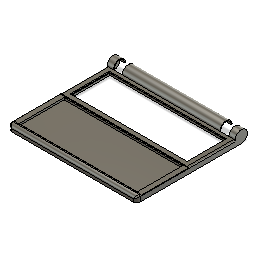
C_case (Autodesk Fusion 360 design; units mm, degrees)
Autodesk Fusion 360 part; units mm, degrees
sketch "Sketch1" plane through (0, 0, 0) normal (0, 1, 0) x (1, 0, 0)
  line L0 (0, 0) -> (230.6, 0)
  line L1 (230.6, 0) -> (230.6, 177.2)
  line L2 (230.6, 177.2) -> (0, 177.2)
  line L3 (0, 177.2) -> (0, 0)
  dimension "d1" = 230.6
  dimension "d2" = 177.2
  constraint horizontal L0
  constraint vertical L1
  constraint horizontal L2
  constraint vertical L3
  constraint coincident L0.start L3.end
  measures "d1" distance of L0.start L0.end
  measures "d2" distance of L0.start L2.end
extrude "Extrude1" add sketch "Sketch1" along normal blind 11 makes body 1
fillet "Fillet3" radius 2.5 2 edges at (230.6, 11, -88.6) (0, 11, -88.6) on bodies 1
sketch "Sketch2" plane through (0, 11, 0) normal (0, 1, 0) x (-1, 0, 0)
  line L0 (-2.5, 0) -> (-228.1, 0)
  line L1 (-228.1, -177.2) -> (-2.5, -177.2)
  line L2 (-9, -10) -> (-221.6, -10)
  line L3 (-221.6, -10) -> (-221.6, -91.1)
  line L4 (-221.6, -91.1) -> (-9, -91.1)
  line L5 (-9, -91.1) -> (-9, -10)
  line L6 (-115.3, -77.3448) -> (-115.3, -22.2714) construction
  line L7 (-228.1, 0) -> (-228.1, -177.2)
  line L8 (-2.5, -177.2) -> (-2.5, 0)
  dimension "d5" = 212.6
  dimension "d6" = 81.1
  dimension "d7" = 10
  constraint horizontal L2
  constraint vertical L3
  constraint horizontal L4
  constraint vertical L5
  constraint perpendicular L1 L6
  constraint symmetric L3 L5 L6
  measures "d5" distance of L3.end L4.end
  measures "d6" distance of L2.start L4.end
  measures "d7" distance of L0 L2
extrude "Extrude2" cut sketch "Sketch2" against normal blind 5 contours L2 L3 L4 L5 bodies 1
sketch "Sketch3" plane through (0, 11, 0) normal (0, 1, 0) x (-1, 0, 0)
  line L0 (-221.6, -10) -> (-9, -10)
  line L1 (-9, -10) -> (-9, -91.1)
  line L2 (-9, -91.1) -> (-221.6, -91.1)
  line L3 (-221.6, -91.1) -> (-221.6, -10)
  line L4 (-2.5, 0) -> (-228.1, 0)
  line L5 (-228.1, -177.2) -> (-2.5, -177.2)
  line L6 (-10.05, -171.2) -> (-220.55, -171.2)
  line L7 (-220.55, -171.2) -> (-220.55, -100.7)
  line L8 (-220.55, -100.7) -> (-10.05, -100.7)
  line L9 (-10.05, -100.7) -> (-10.05, -171.2)
  line L10 (-115.3, -155) -> (-115.3, -110) construction
  line L11 (-228.1, 0) -> (-228.1, -177.2)
  line L12 (-2.5, -177.2) -> (-2.5, 0)
  dimension "d10" = 210.5
  dimension "d11" = 70.5
  dimension "d12" = 6
  constraint horizontal L6
  constraint vertical L7
  constraint horizontal L8
  constraint vertical L9
  constraint vertical L10
  constraint symmetric L7 L9 L10
  measures "d10" distance of L6.start L6.end
  measures "d11" distance of L6.start L8.end
  measures "d12" distance of L5 L6
extrude "Extrude3" cut sketch "Sketch3" against normal blind 1.95 contours L6 L7 L8 L9 bodies 1
sketch "Sketch4" plane through (0, 9.05, 0) normal (0, 1, 0) x (-1, 0, 0)
  line L0 (-10.05, -100.7) -> (-220.55, -100.7)
  line L1 (-220.55, -100.7) -> (-220.55, -171.2)
  line L2 (-220.55, -171.2) -> (-10.05, -171.2)
  line L3 (-10.05, -171.2) -> (-10.05, -100.7)
  line L4 (-11.55, -170.7) -> (-219.05, -170.7)
  line L5 (-219.05, -170.7) -> (-219.05, -101.2)
  line L6 (-219.05, -101.2) -> (-11.55, -101.2)
  line L7 (-11.55, -101.2) -> (-11.55, -170.7)
  dimension "d15" = 0.5
  dimension "d16" = 0.5
  dimension "d17" = 1.5
  dimension "d18" = 1.5
  constraint horizontal L4
  constraint vertical L5
  constraint horizontal L6
  constraint vertical L7
  measures "d15" distance of L2 L4
  measures "d16" distance of L0 L6
  measures "d17" distance of L3 L7
  measures "d18" distance of L1 L5
extrude "Extrude4" cut sketch "Sketch4" against normal blind 4.75 contours L4 L5 L6 L7 bodies 1
sketch "Sketch6" plane through (0, 0, 0) normal (-1, 0, 0) x (0, 0, 1)
  line L0 (-177.2, 0) -> (0, 0)
  line L1 (0, 0) -> (0, 8.5)
  line L2 (-177.2, 8.5) -> (-177.2, 0)
  line L3 (-8, 11) -> (-93, 11)
  line L4 (-93, 11) -> (-93, 9.5)
  line L5 (-93, 9.5) -> (-8, 9.5)
  line L6 (-8, 9.5) -> (-8, 11)
  line L7 (0, 8.5) -> (-177.2, 8.5)
  dimension "d26" = 1.5
  dimension "d27" = 85
  dimension "d28" = 8
  constraint horizontal L3
  constraint vertical L4
  constraint horizontal L5
  constraint vertical L6
  measures "d26" distance of L3.start L5.end
  measures "d27" distance of L3.start L3.end
  measures "d28" distance of L1 L6
extrude "Extrude6" cut sketch "Sketch6" against normal through all contours L3 L4 L5 L6 bodies 1
sketch "Sketch7" plane through (0, 6, 0) normal (0, 1, 0) x (-1, 0, 0)
  line L0 (-9, -91.1) -> (-9, -10)
  line L1 (-9, -10) -> (-221.6, -10)
  line L2 (-221.6, -10) -> (-221.6, -91.1)
  line L3 (-221.6, -91.1) -> (-9, -91.1)
  line L4 (-54, -11.5) -> (-92, -11.5)
  line L5 (-92, -11.5) -> (-92, -23.5)
  line L6 (-92, -23.5) -> (-54, -23.5)
  line L7 (-54, -23.5) -> (-54, -11.5)
  dimension "d32" = 38
  dimension "d33" = 12
  dimension "d34" = 45
  dimension "d35" = 1.5
  constraint horizontal L4
  constraint vertical L5
  constraint horizontal L6
  constraint vertical L7
  measures "d32" distance of L5.end L6.end
  measures "d33" distance of L4.end L5.end
  measures "d34" distance of L0 L7
  measures "d35" distance of L1 L4
sketch "Sketch8" plane through (0, 0, 0) normal (-1, 0, 0) x (0, 0, 1)
  line L0 (-177.2, 8.5) -> (-177.2, 0)
  line L1 (-177.2, 0) -> (0, 0)
  line L2 (0, 0) -> (0, 8.5)
  circle A0 centre (-188.2, 11) radius 11
  circle A1 centre (-188.2, 11) radius 9.5
  line L3 (-177.2, 0) -> (-188.2, 0)
  line L4 (0, 8.5) -> (-177.2, 8.5)
  line L5 (-177.2, 0) -> (-177.2, 11)
  dimension "d36" = 22
  dimension "d37" = 19
  constraint tangent L0 A0
  constraint concentric A0 A1
  constraint coincident L0.end L1.start
  constraint coincident A0 L3.end
  constraint tangent A0 L3
  constraint parallel L1 L3
  constraint coincident A0 L5.end
  constraint tangent A0 L5
  measures "d36" diameter of A0
  measures "d37" diameter of A1
extrude "Extrude7" add sketch "Sketch8" against normal blind 230.6 separate body contours A0 makes body 2
extrude "Extrude8" add sketch "Sketch8" against normal blind 1.5 contours L0 A0 L3 L5 | A0 | A1 bodies 2 1
sketch "Sketch9" plane through (230.6, 0, 0) normal (1, 0, 0) x (0, 0, -1)
  circle A0 centre (188.2, 11) radius 9.5
  circle A1 centre (188.2, 11) radius 11
  circle A2 centre (188.2, 11) radius 11
  line L0 (177.2, 0) -> (188.2, 0)
  line L1 (177.2, 0) -> (188.2, 0)
  line L2 (177.2, 0) -> (177.2, 8.5)
  line L3 (177.2, 0) -> (177.2, 11)
  point P0 (177.2, 8.5)
  constraint concentric A0 A2
  constraint coincident A1 L0.end
  constraint tangent A1 L0
  constraint parallel L0 L1
  constraint coincident L0.start L1.start
  constraint coincident P0 L2.end
  constraint coincident A2 L0.end
  constraint coincident A2 L3.end
  constraint tangent A2 L3
extrude "Extrude9" add sketch "Sketch9" against normal blind 1.5 contours A0 | A1 A2 | A1 A2 L0 L1 L2 L3 bodies 2
sketch "Sketch5" plane through (0, 0, 0) normal (0, -1, 0) x (1, 0, 0)
  line L0 (0, 0) -> (0, -188.2)
  line L1 (1.5, -177.2) -> (229.1, -177.2)
  line L2 (230.6, -188.2) -> (230.6, 0)
  line L3 (230.6, 0) -> (0, 0)
  line L4 (1.5, -177.2) -> (229.1, -177.2)
  line L5 (229.1, -177.2) -> (229.1, -3.5)
  line L6 (229.1, -3.5) -> (1.5, -3.5)
  line L7 (1.5, -3.5) -> (1.5, -177.2)
  line L8 (1.5, -177.2) -> (229.1, -177.2)
  line L9 (229.1, -177.2) -> (229.1, -199.2)
  line L10 (229.1, -199.2) -> (1.5, -199.2)
  line L11 (1.5, -199.2) -> (1.5, -177.2)
  line L12 (0, -188.2) -> (1.5, -188.2)
  line L13 (1.5, -188.2) -> (1.5, -177.2)
  line L14 (229.1, -177.2) -> (229.1, -188.2)
  line L15 (229.1, -188.2) -> (230.6, -188.2)
  line L16 (219.1, -177.2) -> (203.1, -177.2)
  line L17 (203.1, -177.2) -> (203.1, -199.2)
  line L18 (203.1, -199.2) -> (219.1, -199.2)
  line L19 (219.1, -199.2) -> (219.1, -177.2)
  line L20 (11.5, -177.2) -> (27.5, -177.2)
  line L21 (27.5, -177.2) -> (27.5, -199.2)
  line L22 (27.5, -199.2) -> (11.5, -199.2)
  line L23 (11.5, -199.2) -> (11.5, -177.2)
  dimension "d21" = 1.5
  dimension "d22" = 1.5
  dimension "d23" = 3.5
  dimension "d44" = 22
  dimension "d51" = 10
  dimension "d52" = 16
  dimension "d53" = 10
  dimension "d54" = 16
  constraint horizontal L4
  constraint vertical L5
  constraint horizontal L6
  constraint vertical L7
  constraint coincident L1 L4.start
  constraint horizontal L8
  constraint vertical L9
  constraint horizontal L10
  constraint vertical L11
  constraint coincident L1.start L4.start
  constraint collinear L5 L9
  constraint horizontal L16
  constraint vertical L17
  constraint horizontal L18
  constraint vertical L19
  constraint coincident L10 L17.end
  constraint coincident L4 L16.start
  constraint horizontal L20
  constraint vertical L21
  constraint horizontal L22
  constraint vertical L23
  constraint coincident L10 L21.end
  constraint coincident L4 L20.start
  measures "d21" distance of L0 L7
  measures "d22" distance of L2 L5
  measures "d23" distance of L3 L6
  measures "d44" distance of L1.end L9.end
  measures "d51" distance of L11 L23
  measures "d52" distance of L21.end L22.end
  measures "d53" distance of L9 L19
  measures "d54" distance of L17 L19
extrude "Extrude5" cut sketch "Sketch5" against normal blind 5.4 contours L1 L4 L5 L6 L7 L8 L16 L20 bodies 2
extrude "Extrude10" cut sketch "Sketch5" against normal blind 11 contours L1 L4 L8 L10 L11 L13 L23 | L1 L4 L8 L9 L10 L14 L19 | L1 L4 L8 L10 L20 L21 L22 L23 | L1 L4 L8 L10 L17 L21 | L1 L4 L8 L10 L16 L17 L18 L19 bodies 2
fillet "Fillet1" radius 6 5 edges at (115.3, 11, 0) (229.8678, 10.2678, 0) (230.6, 4.25, 0) (0.7322, 10.2678, 0) (0, 4.25, 0) on bodies 2
extrude "Extrude11" cut sketch "Sketch5" against normal through all contours L1 L4 L8 L10 L20 L21 L22 L23 | L1 L4 L8 L10 L16 L17 L18 L19 bodies 2
